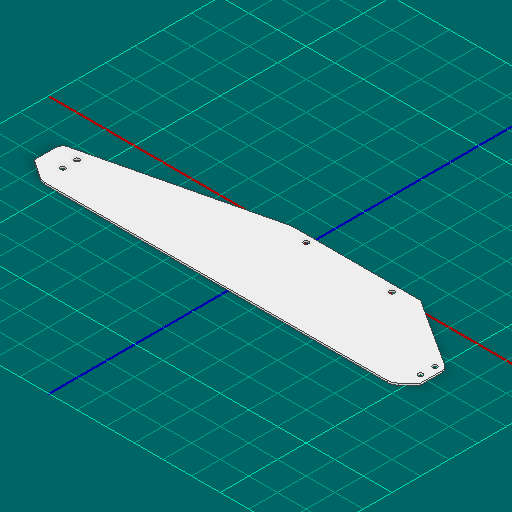
# Autodesk Inventor part: skirt
Saved by Autodesk Inventor 2025 (Build 290162000, 162)
## iProperties
Created: 2024-08-23
Part Number: skirt
Material: Acetal Resin, White
Document SubType Name: Modeling
Designer: averey
Density: 1.425 g/cm^3
Appearance: Smooth - White
Author: averey
Autodesk Inventor part; units mm, degrees
ref_plane "YZ Plane" through (0, 0, 0) normal (1, 0, 0) x (0, 1, 0)
ref_plane "XZ Plane" through (0, 0, 0) normal (0, 1, 0) x (-1, 0, 0)
ref_plane "XY Plane" through (0, 0, 0) normal (0, 0, 1) x (1, 0, 0)
sketch "main" plane through (0, 0, 0) normal (0, 0, 1) x (1, 0, 0)
  circle A0 centre (45.9011, -170.4057) radius 2.1844
  circle A1 centre (58.6011, -170.4057) radius 2.1844
  arc A2 (39.5511, -183.1057) -> (45.9011, -189.4557) centre (45.9011, -183.1057) ccw
  line L0 (45.9011, -189.4557) -> (58.6011, -189.4557)
  line L1 (39.5511, -183.1057) -> (1.4511, -24.3557)
  arc A3 (76.0514, -172.8053) -> (77.6511, -167.5218) centre (68.1261, -167.5218) ccw
  line L2 (64.9511, -189.4557) -> (76.0514, -172.8053)
  line L3 (58.6011, -189.4557) -> (64.9511, -189.4557)
  circle A4 centre (45.9011, 147.0943) radius 2.1844
  circle A5 centre (58.6011, 147.0943) radius 2.1844
  circle A6 centre (7.8011, -5.3057) radius 2.1844
  circle A7 centre (7.8011, 70.8943) radius 2.1844
  line L4 (77.6511, -167.5218) -> (77.6511, 136.7989)
  line L5 (1.4511, -24.3557) -> (1.4511, 89.9443)
  arc A8 (77.6511, 136.7989) -> (74.8613, 143.5341) centre (68.1261, 136.7989) ccw
  line L6 (74.8613, 143.5341) -> (64.9511, 153.4443)
  line L7 (64.9511, 153.4443) -> (58.6011, 153.4443)
  line L8 (45.9011, 153.4443) -> (58.6011, 153.4443)
  arc A9 (45.9011, 153.4443) -> (40.5661, 150.5382) centre (45.9011, 147.0943) ccw
  line L9 (1.4511, 89.9443) -> (40.5661, 150.5382)
  point P0 (53.0582, -9.4982)
  point P1 (77.6511, -170.4057)
  point P2 (77.6511, -189.4557)
  point P3 (77.6511, 140.7443)
  point P4 (77.6511, 153.4443)
  dimension "d0" = 19.05
  dimension "d1" = 12.7
  dimension "d2" = 19.05
  dimension "d3" = 12.7
  dimension "d4" = 12.7
  dimension "d5" = 19.05
  dimension "d6" = 9.525
  measures "d0" distance of L0.end point (77.651, -189.456)
  measures "d1" distance of L3.end point (77.651, -189.456)
  measures "d2" distance of point (77.651, -170.406) point (77.651, -189.456)
  measures "d3" distance of point (77.651, 140.744) point (77.651, 153.444)
  measures "d4" distance of L7.start point (77.651, 153.444)
  measures "d5" distance of L0.start L3.end
  measures "d6" radius of A3
sketch "Sketch1" plane through (0, 0, 0) normal (0, 1, 0) x (-1, 0, 0)
  circle A0 centre (165.1067, 38.0709) radius 2.1844
  circle A1 centre (165.109, 50.7709) radius 2.1844
  arc A2 (177.8056, 31.7187) -> (184.1567, 38.0675) centre (177.8067, 38.0687) ccw
  line L0 (184.1567, 38.0675) -> (184.159, 50.7675)
  line L1 (177.8056, 31.7187) -> (19.0489, -6.3534)
  arc A3 (167.5116, 68.2207) -> (162.2284, 69.8214) centre (162.2267, 60.2964) ccw
  line L2 (184.1601, 57.1175) -> (167.5116, 68.2207)
  line L3 (184.159, 50.7675) -> (184.1601, 57.1175)
  circle A4 centre (-152.3933, 38.1269) radius 2.1844
  circle A5 centre (-152.391, 50.8269) radius 2.1844
  circle A6 centre (0, 0) radius 2.1844
  circle A7 centre (-76.2, 0.0134) radius 2.1844
  line L4 (162.2284, 69.8214) -> (-142.0923, 69.8751)
  line L5 (19.0489, -6.3534) -> (-95.2511, -6.3332)
  arc A8 (-142.0923, 69.8751) -> (-148.828, 67.0864) centre (-142.094, 60.3501) ccw
  line L6 (-148.828, 67.0864) -> (-158.7399, 57.178)
  line L7 (-158.7399, 57.178) -> (-158.741, 50.828)
  line L8 (-158.7433, 38.128) -> (-158.741, 50.828)
  arc A9 (-158.7433, 38.128) -> (-155.8381, 32.7925) centre (-152.3933, 38.1269) ccw
  line L9 (-95.2511, -6.3332) -> (-155.8381, 32.7925)
  point P0 (0, 0)
  constraints: 1 other
extrude "Extrusion1" add sketch "Sketch1" along normal blind 1.5875
equation "\"d4\" = d3"
body "Solid1"
